Autodesk Fusion 360 part; units mm, degrees
note: some values were not read from the file. Set by a fixed rule: which sketch regions a step uses.
(part 4 of 5)
  line L709 (-95.6805, -65.95) -> (-95.5765, -65.8721)
  line L710 (-95.5765, -65.8721) -> (-95.4672, -65.8024)
  line L711 (-95.4672, -65.8024) -> (-95.3531, -65.7412)
  line L712 (-95.3531, -65.7412) -> (-95.2348, -65.6887)
  line L713 (-95.2348, -65.6887) -> (-95.1128, -65.6452)
  line L714 (-95.1128, -65.6452) -> (-94.9876, -65.6109)
  line L715 (-94.9876, -65.6109) -> (-94.8598, -65.586)
  line L716 (-94.8598, -65.586) -> (-94.7298, -65.5709)
  line L717 (-94.7298, -65.5709) -> (-94.5983, -65.5659)
  line L718 (-94.5983, -65.5659) -> (-94.4542, -65.5719)
  line L719 (-94.4542, -65.5719) -> (-94.3095, -65.5904)
  line L720 (-94.3095, -65.5904) -> (-94.1649, -65.6216)
  line L721 (-94.1649, -65.6216) -> (-94.0212, -65.666)
  line L722 (-94.0212, -65.666) -> (-93.8589, -65.7335)
  line L723 (-93.8589, -65.7335) -> (-93.7072, -65.8154)
  line L724 (-93.7072, -65.8154) -> (-93.5666, -65.9106)
  line L725 (-93.5666, -65.9106) -> (-93.4375, -66.0181)
  line L726 (-93.4375, -66.0181) -> (-93.3205, -66.1366)
  line L727 (-93.3205, -66.1366) -> (-93.2162, -66.2652)
  line L728 (-93.2162, -66.2652) -> (-93.125, -66.4027)
  line L729 (-93.125, -66.4027) -> (-93.0475, -66.548)
  line L730 (-93.0475, -66.548) -> (-92.9842, -66.7)
  line L731 (-92.9842, -66.7) -> (-92.9356, -66.8576)
  line L732 (-92.9356, -66.8576) -> (-92.9022, -67.0198)
  line L733 (-92.9022, -67.0198) -> (-92.8846, -67.1853)
  line L734 (-92.8846, -67.1853) -> (-92.8836, -67.3531)
  line L735 (-92.8836, -67.3531) -> (-92.8991, -67.5221)
  line L736 (-92.8991, -67.5221) -> (-92.9319, -67.6912)
  line L737 (-92.9319, -67.6912) -> (-92.9826, -67.8593)
  line L738 (-92.9826, -67.8593) -> (-95.8873, -75.988)
  line L739 (-95.8873, -75.988) -> (-94.5986, -75.988)
  line L740 (-94.5986, -75.988) -> (-94.479, -75.994)
  line L741 (-94.479, -75.994) -> (-94.3628, -76.0117)
  line L742 (-94.3628, -76.0117) -> (-94.2506, -76.0405)
  line L743 (-94.2506, -76.0405) -> (-94.1431, -76.0799)
  line L744 (-94.1431, -76.0799) -> (-94.0408, -76.1291)
  line L745 (-94.0408, -76.1291) -> (-93.9443, -76.1877)
  line L746 (-93.9443, -76.1877) -> (-93.8542, -76.2551)
  line L747 (-93.8542, -76.2551) -> (-93.7711, -76.3306)
  line L748 (-93.7711, -76.3306) -> (-93.6955, -76.4137)
  line L749 (-93.6955, -76.4137) -> (-93.6281, -76.5038)
  line L750 (-93.6281, -76.5038) -> (-93.5695, -76.6003)
  line L751 (-93.5695, -76.6003) -> (-93.5202, -76.7026)
  line L752 (-93.5202, -76.7026) -> (-93.4808, -76.8102)
  line L753 (-93.4808, -76.8102) -> (-93.4519, -76.9224)
  line L754 (-93.4519, -76.9224) -> (-93.4342, -77.0387)
  line L755 (-93.4342, -77.0387) -> (-93.4282, -77.1585)
  line L756 (-93.4282, -77.1585) -> (-93.4342, -77.2781)
  line L757 (-93.4342, -77.2781) -> (-93.4519, -77.3943)
  line L758 (-93.4519, -77.3943) -> (-93.4808, -77.5065)
  line L759 (-93.4808, -77.5065) -> (-93.5202, -77.614)
  line L760 (-93.5202, -77.614) -> (-93.5695, -77.7163)
  line L761 (-93.5695, -77.7163) -> (-93.6281, -77.8128)
  line L762 (-93.6281, -77.8128) -> (-93.6955, -77.9029)
  line L763 (-93.6955, -77.9029) -> (-93.7711, -77.986)
  line L764 (-93.7711, -77.986) -> (-93.8542, -78.0616)
  line L765 (-93.8542, -78.0616) -> (-93.9443, -78.129)
  line L766 (-93.9443, -78.129) -> (-94.0408, -78.1876)
  line L767 (-94.0408, -78.1876) -> (-94.1431, -78.2369)
  line L768 (-94.1431, -78.2369) -> (-94.2506, -78.2763)
  line L769 (-94.2506, -78.2763) -> (-94.3628, -78.3051)
  line L770 (-94.3628, -78.3051) -> (-94.479, -78.3229)
  line L771 (-94.479, -78.3229) -> (-94.5986, -78.3289)
  line L772 (-94.5986, -78.3289) -> (-98.0467, -78.3289)
  line L773 (-98.0467, -78.3289) -> (-98.1858, -78.3189)
  line L774 (-98.1858, -78.3189) -> (-98.3201, -78.293)
  line L775 (-98.3201, -78.293) -> (-98.4083, -78.3)
  line L776 (-98.4083, -78.3) -> (-98.4224, -78.299)
  line L777 (-98.4224, -78.299) -> (-98.606, -78.291)
  line L778 (-98.606, -78.291) -> (-98.7865, -78.2694)
  line L779 (-98.7865, -78.2694) -> (-98.9634, -78.2348)
  line L780 (-98.9634, -78.2348) -> (-99.1359, -78.1876)
  line L781 (-99.1359, -78.1876) -> (-99.3035, -78.1282)
  line L782 (-99.3035, -78.1282) -> (-99.4654, -78.0571)
  line L783 (-99.4654, -78.0571) -> (-99.6212, -77.9746)
  line L784 (-99.6212, -77.9746) -> (-99.7701, -77.8812)
  line L785 (-99.7701, -77.8812) -> (-99.9116, -77.7774)
  line L786 (-99.9116, -77.7774) -> (-100.045, -77.6636)
  line L787 (-100.045, -77.6636) -> (-100.1696, -77.5402)
  line L788 (-100.1696, -77.5402) -> (-100.285, -77.4076)
  line L789 (-100.285, -77.4076) -> (-100.3903, -77.2662)
  line L790 (-100.3903, -77.2662) -> (-100.4851, -77.1166)
  line L791 (-100.4851, -77.1166) -> (-100.5686, -76.959)
  line L792 (-100.5686, -76.959) -> (-100.6403, -76.7941)
  line L793 (-100.6403, -76.7941) -> (-102.7545, -71.7649)
  line L794 (-102.7545, -71.7649) -> (-104.868, -76.793)
  line L795 (-104.868, -76.793) -> (-104.9397, -76.9586)
  line L796 (-104.9397, -76.9586) -> (-105.0233, -77.1168)
  line L797 (-105.0233, -77.1168) -> (-105.1182, -77.267)
  line L798 (-105.1182, -77.267) -> (-105.2238, -77.4089)
  line L799 (-105.2238, -77.4089) -> (-105.3395, -77.542)
  line L800 (-105.3395, -77.542) -> (-105.4645, -77.6658)
  line L801 (-105.4645, -77.6658) -> (-105.5984, -77.78)
  line L802 (-105.5984, -77.78) -> (-105.7403, -77.8841)
  line L803 (-105.7403, -77.8841) -> (-105.8898, -77.9776)
  line L804 (-105.8898, -77.9776) -> (-106.0461, -78.0602)
  line L805 (-106.0461, -78.0602) -> (-106.2087, -78.1313)
  line L806 (-106.2087, -78.1313) -> (-106.3768, -78.1906)
  line L807 (-106.3768, -78.1906) -> (-106.5499, -78.2376)
  line L808 (-106.5499, -78.2376) -> (-106.7273, -78.2719)
  line L809 (-106.7273, -78.2719) -> (-106.9084, -78.293)
  line L810 (-106.9084, -78.293) -> (-107.0926, -78.3)
  line L811 (-107.0926, -78.3) -> (-107.0996, -78.3008)
  line L812 (-107.0996, -78.3008) -> (-107.288, -78.2938)
  line L813 (-107.288, -78.2938) -> (-107.4733, -78.2722)
  line L814 (-107.4733, -78.2722) -> (-107.6547, -78.2368)
  line L815 (-107.6547, -78.2368) -> (-107.8316, -78.1881)
  line L816 (-107.8316, -78.1881) -> (-108.0032, -78.1266)
  line L817 (-108.0032, -78.1266) -> (-108.169, -78.0527)
  line L818 (-108.169, -78.0527) -> (-108.3282, -77.9669)
  line L819 (-108.3282, -77.9669) -> (-108.4802, -77.8696)
  line L820 (-108.4802, -77.8696) -> (-108.6242, -77.7613)
  line L821 (-108.6242, -77.7613) -> (-108.7595, -77.6426)
  line L822 (-108.7595, -77.6426) -> (-108.8856, -77.5138)
  line L823 (-108.8856, -77.5138) -> (-109.0017, -77.3755)
  line L824 (-109.0017, -77.3755) -> (-109.1071, -77.2281)
  line L825 (-109.1071, -77.2281) -> (-109.2012, -77.0721)
  line L826 (-109.2012, -77.0721) -> (-109.2832, -76.9079)
  line L827 (-109.2832, -76.9079) -> (-109.3525, -76.7362)
  line L828 (-109.3525, -76.7362) -> (-112.5246, -67.8603)
  line L829 (-112.5246, -67.8603) -> (-112.5744, -67.6917)
  line L830 (-112.5744, -67.6917) -> (-112.6072, -67.5226)
  line L831 (-112.6072, -67.5226) -> (-112.6227, -67.3536)
  line L832 (-123.9451, -66.3953) -> (-123.8658, -66.5621)
  line L833 (-123.8658, -66.5621) -> (-123.8011, -66.7379)
  line L834 (-123.8011, -66.7379) -> (-123.7502, -66.9213)
  line L835 (-123.7502, -66.9213) -> (-123.7123, -67.1111)
  line L836 (-123.7123, -67.1111) -> (-123.6866, -67.3062)
  line L837 (-123.6866, -67.3062) -> (-123.6722, -67.5054)
  line L838 (-123.6722, -67.5054) -> (-123.4156, -67.2357)
  line L839 (-123.4156, -67.2357) -> (-123.1539, -66.9883)
  line L840 (-123.1539, -66.9883) -> (-122.887, -66.7624)
  line L841 (-122.887, -66.7624) -> (-122.6149, -66.5573)
  line L842 (-122.6149, -66.5573) -> (-122.3375, -66.3725)
  line L843 (-122.3375, -66.3725) -> (-122.0547, -66.2072)
  line L844 (-122.0547, -66.2072) -> (-121.7664, -66.0609)
  line L845 (-121.7664, -66.0609) -> (-121.4727, -65.9327)
  line L846 (-121.4727, -65.9327) -> (-121.1733, -65.8221)
  line L847 (-121.1733, -65.8221) -> (-120.8684, -65.7284)
  line L848 (-120.8684, -65.7284) -> (-120.5577, -65.6509)
  line L849 (-120.5577, -65.6509) -> (-120.2412, -65.589)
  line L850 (-120.2412, -65.589) -> (-119.9188, -65.542)
  line L851 (-119.9188, -65.542) -> (-119.5906, -65.5093)
  line L852 (-119.5906, -65.5093) -> (-119.2563, -65.4903)
  line L853 (-119.2563, -65.4903) -> (-118.916, -65.4843)
  line L854 (-118.916, -65.4843) -> (-118.7311, -65.4883)
  line L855 (-118.7311, -65.4883) -> (-118.5467, -65.5002)
  line L856 (-118.5467, -65.5002) -> (-118.3631, -65.5198)
  line L857 (-118.3631, -65.5198) -> (-118.1807, -65.547)
  line L858 (-118.1807, -65.547) -> (-117.9999, -65.5818)
  line L859 (-117.9999, -65.5818) -> (-117.8209, -65.624)
  line L860 (-117.8209, -65.624) -> (-117.6443, -65.6736)
  line L861 (-117.6443, -65.6736) -> (-117.4702, -65.7305)
  line L862 (-117.4702, -65.7305) -> (-117.2991, -65.7945)
  line L863 (-117.2991, -65.7945) -> (-117.1313, -65.8656)
  line L864 (-117.1313, -65.8656) -> (-116.9672, -65.9437)
  line L865 (-116.9672, -65.9437) -> (-116.8071, -66.0287)
  line L866 (-116.8071, -66.0287) -> (-116.6513, -66.1205)
  line L867 (-116.6513, -66.1205) -> (-116.5003, -66.219)
  line L868 (-116.5003, -66.219) -> (-116.3544, -66.3241)
  line L869 (-116.3544, -66.3241) -> (-116.2139, -66.4357)
  line L870 (-116.2139, -66.4357) -> (-116.0791, -66.5536)
  line L871 (-116.0791, -66.5536) -> (-115.9505, -66.6779)
  line L872 (-115.9505, -66.6779) -> (-115.8284, -66.8085)
  line L873 (-115.8284, -66.8085) -> (-115.7132, -66.9451)
  line L874 (-115.7132, -66.9451) -> (-115.6051, -67.0878)
  line L875 (-115.6051, -67.0878) -> (-115.5046, -67.2364)
  line L876 (-115.5046, -67.2364) -> (-115.412, -67.3908)
  line L877 (-115.412, -67.3908) -> (-115.3276, -67.551)
  line L878 (-115.3276, -67.551) -> (-115.2518, -67.7168)
  line L879 (-115.2518, -67.7168) -> (-115.185, -67.8882)
  line L880 (-115.185, -67.8882) -> (-115.1275, -68.065)
  line L881 (-115.1275, -68.065) -> (-115.0797, -68.2472)
  line L882 (-115.0797, -68.2472) -> (-115.0419, -68.4346)
  line L883 (-115.0419, -68.4346) -> (-115.0145, -68.6272)
  line L884 (-115.0145, -68.6272) -> (-114.9978, -68.8249)
  line L885 (-114.9978, -68.8249) -> (-114.9918, -69.0276)
  line L886 (-114.9918, -69.0276) -> (-114.9978, -69.2913)
  line L887 (-114.9978, -69.2913) -> (-115.0167, -69.5432)
  line L888 (-115.0167, -69.5432) -> (-115.0478, -69.7836)
  line L889 (-115.0478, -69.7836) -> (-115.0907, -70.0127)
  line L890 (-115.0907, -70.0127) -> (-115.1452, -70.2308)
  line L891 (-115.1452, -70.2308) -> (-115.2109, -70.4382)
  line L892 (-115.2109, -70.4382) -> (-115.2876, -70.6352)
  line L893 (-115.2876, -70.6352) -> (-115.3749, -70.8221)
  line L894 (-115.3749, -70.8221) -> (-115.4725, -70.9992)
  line L895 (-115.4725, -70.9992) -> (-115.5801, -71.1668)
  line L896 (-115.5801, -71.1668) -> (-115.6974, -71.3251)
  line L897 (-115.6974, -71.3251) -> (-115.8241, -71.4744)
  line L898 (-115.8241, -71.4744) -> (-115.9599, -71.6151)
  line L899 (-115.9599, -71.6151) -> (-116.1043, -71.7474)
  line L900 (-116.1043, -71.7474) -> (-116.2573, -71.8716)
  line L901 (-116.2573, -71.8716) -> (-116.4183, -71.9879)
  line L902 (-116.4183, -71.9879) -> (-116.5871, -72.0968)
  line L903 (-116.5871, -72.0968) -> (-116.7634, -72.1984)
  line L904 (-116.7634, -72.1984) -> (-116.9469, -72.2931)
  line L905 (-116.9469, -72.2931) -> (-117.1373, -72.3811)
  line L906 (-117.1373, -72.3811) -> (-117.3342, -72.4627)
  line L907 (-117.3342, -72.4627) -> (-117.5374, -72.5382)
  line L908 (-117.5374, -72.5382) -> (-117.9611, -72.6722)
  line L909 (-117.9611, -72.6722) -> (-118.406, -72.7853)
  line L910 (-118.406, -72.7853) -> (-118.8696, -72.8798)
  line L911 (-118.8696, -72.8798) -> (-119.3494, -72.958)
  line L912 (-119.3494, -72.958) -> (-119.8428, -73.0222)
  line L913 (-119.8428, -73.0222) -> (-119.9037, -73.0252)
  line L914 (-119.9037, -73.0252) -> (-120.0568, -73.0282)
  line L915 (-120.0568, -73.0282) -> (-120.2756, -73.0155)
  line L916 (-120.2756, -73.0155) -> (-120.4012, -72.9983)
  line L917 (-120.4012, -72.9983) -> (-120.5332, -72.9709)
  line L918 (-120.5332, -72.9709) -> (-120.6684, -72.9315)
  line L919 (-120.6684, -72.9315) -> (-120.8032, -72.878)
  line L920 (-120.8032, -72.878) -> (-120.9345, -72.8083)
  line L921 (-120.9345, -72.8083) -> (-121.0588, -72.7204)
  line L922 (-121.0588, -72.7204) -> (-121.1729, -72.6123)
  line L923 (-121.1729, -72.6123) -> (-121.2734, -72.482)
  line L924 (-121.2734, -72.482) -> (-121.357, -72.3274)
  line L925 (-121.357, -72.3274) -> (-121.4203, -72.1465)
  line L926 (-121.4203, -72.1465) -> (-121.4581, -71.9616)
  line L927 (-121.4581, -71.9616) -> (-121.4694, -71.7956)
  line L928 (-121.4694, -71.7956) -> (-121.4576, -71.6475)
  line L929 (-121.4576, -71.6475) -> (-121.4259, -71.5165)
  line L930 (-121.4259, -71.5165) -> (-121.3776, -71.4014)
  line L931 (-121.3776, -71.4014) -> (-121.3161, -71.3013)
  line L932 (-121.3161, -71.3013) -> (-121.2446, -71.2152)
  line L933 (-121.2446, -71.2152) -> (-121.1665, -71.1421)
  line L934 (-121.1665, -71.1421) -> (-121.0851, -71.081)
  line L935 (-121.0851, -71.081) -> (-121.0036, -71.031)
  line L936 (-121.0036, -71.031) -> (-120.8538, -70.9601)
  line L937 (-120.8538, -70.9601) -> (-120.7434, -70.9215)
  line L938 (-120.7434, -70.9215) -> (-120.6989, -70.9072)
  line L939 (-120.6989, -70.9072) -> (-120.4347, -70.8642)
  line L940 (-120.4347, -70.8642) -> (-120.1863, -70.8151)
  line L941 (-120.1863, -70.8151) -> (-119.9539, -70.7594)
  line L942 (-119.9539, -70.7594) -> (-119.7376, -70.6965)
  line L943 (-119.7376, -70.6965) -> (-119.5376, -70.6259)
  line L944 (-119.5376, -70.6259) -> (-119.354, -70.5472)
  line L945 (-119.354, -70.5472) -> (-119.1872, -70.4597)
  line L946 (-119.1872, -70.4597) -> (-119.0371, -70.363)
  line L947 (-119.0371, -70.363) -> (-118.9041, -70.2565)
  line L948 (-118.9041, -70.2565) -> (-118.7882, -70.1398)
  line L949 (-118.7882, -70.1398) -> (-118.6897, -70.0123)
  line L950 (-118.6897, -70.0123) -> (-118.6087, -69.8735)
  line L951 (-118.6087, -69.8735) -> (-118.5454, -69.7228)
  line L952 (-118.5454, -69.7228) -> (-118.5, -69.5598)
  line L953 (-118.5, -69.5598) -> (-118.4726, -69.384)
  line L954 (-118.4726, -69.384) -> (-118.4636, -69.1947)
  line L955 (-118.4636, -69.1947) -> (-118.4726, -69.0494)
  line L956 (-118.4726, -69.0494) -> (-118.4981, -68.9082)
  line L957 (-118.4981, -68.9082) -> (-118.54, -68.7717)
  line L958 (-118.54, -68.7717) -> (-118.5979, -68.6408)
  line L959 (-118.5979, -68.6408) -> (-118.6715, -68.5162)
  line L960 (-118.6715, -68.5162) -> (-118.7602, -68.3986)
  line L961 (-118.7602, -68.3986) -> (-118.8637, -68.2887)
  line L962 (-118.8637, -68.2887) -> (-118.9816, -68.1873)
  line L963 (-118.9816, -68.1873) -> (-119.1134, -68.0951)
  line L964 (-119.1134, -68.0951) -> (-119.2587, -68.0128)
  line L965 (-119.2587, -68.0128) -> (-119.417, -67.9412)
  line L966 (-119.417, -67.9412) -> (-119.5881, -67.881)
  line L967 (-119.5881, -67.881) -> (-119.7714, -67.8329)
  line L968 (-119.7714, -67.8329) -> (-119.9665, -67.7976)
  line L969 (-119.9665, -67.7976) -> (-120.173, -67.7759)
  line L970 (-120.173, -67.7759) -> (-120.3905, -67.7689)
  line L971 (-120.3905, -67.7689) -> (-120.7384, -67.7832)
  line L972 (-120.7384, -67.7832) -> (-121.0683, -67.8246)
  line L973 (-121.0683, -67.8246) -> (-121.3798, -67.8915)
  line L974 (-121.3798, -67.8915) -> (-121.6721, -67.9822)
  line L975 (-121.6721, -67.9822) -> (-121.9446, -68.0949)
  line L976 (-121.9446, -68.0949) -> (-122.1967, -68.2279)
  line L977 (-122.1967, -68.2279) -> (-122.4278, -68.3793)
  line L978 (-122.4278, -68.3793) -> (-122.6372, -68.5476)
  line L979 (-122.6372, -68.5476) -> (-122.8244, -68.7308)
  line L980 (-122.8244, -68.7308) -> (-122.9886, -68.9274)
  line L981 (-122.9886, -68.9274) -> (-123.1293, -69.1355)
  line L982 (-123.1293, -69.1355) -> (-123.2458, -69.3535)
  line L983 (-123.2458, -69.3535) -> (-123.3375, -69.5795)
  line L984 (-123.3375, -69.5795) -> (-123.4038, -69.8118)
  line L985 (-123.4038, -69.8118) -> (-123.444, -70.0488)
  line L986 (-123.444, -70.0488) -> (-123.4576, -70.2886)
  line L987 (-123.4576, -70.2886) -> (-123.4576, -74.5459)
  line L988 (-123.4576, -74.5459) -> (-123.4458, -74.7233)
  line L989 (-123.4458, -74.7233) -> (-123.4114, -74.8818)
  line L990 (-123.4114, -74.8818) -> (-123.3556, -75.0225)
  line L991 (-123.3556, -75.0225) -> (-123.2797, -75.1463)
  line L992 (-123.2797, -75.1463) -> (-123.185, -75.2544)
  line L993 (-123.185, -75.2544) -> (-123.0728, -75.3477)
  line L994 (-123.0728, -75.3477) -> (-122.9443, -75.4272)
  line L995 (-122.9443, -75.4272) -> (-122.801, -75.494)
  line L996 (-122.801, -75.494) -> (-122.6439, -75.5491)
  line L997 (-122.6439, -75.5491) -> (-122.4745, -75.5935)
  line L998 (-122.4745, -75.5935) -> (-122.294, -75.6283)
  line L999 (-122.294, -75.6283) -> (-122.1036, -75.6545)
  line L1000 (-122.1036, -75.6545) -> (-121.6987, -75.685)
  line L1001 (-121.6987, -75.685) -> (-121.2699, -75.693)
  line L1002 (-121.2699, -75.693) -> (-120.0878, -75.693)
  line L1003 (-120.0878, -75.693) -> (-116.8006, -75.1659)
  line L1004 (-116.8006, -75.1659) -> (-116.6326, -75.1503)
  line L1005 (-116.6326, -75.1503) -> (-116.4755, -75.1533)
  line L1006 (-116.4755, -75.1533) -> (-116.3294, -75.1745)
  line L1007 (-116.3294, -75.1745) -> (-116.1941, -75.2121)
  line L1008 (-116.1941, -75.2121) -> (-116.0697, -75.2646)
  line L1009 (-116.0697, -75.2646) -> (-115.9561, -75.3306)
  line L1010 (-115.9561, -75.3306) -> (-115.8534, -75.4086)
  line L1011 (-115.8534, -75.4086) -> (-115.7616, -75.4972)
  line L1012 (-115.7616, -75.4972) -> (-115.6806, -75.595)
  line L1013 (-115.6806, -75.595) -> (-115.6104, -75.7006)
  line L1014 (-115.6104, -75.7006) -> (-115.551, -75.8125)
  line L1015 (-115.551, -75.8125) -> (-115.5025, -75.9293)
  line L1016 (-115.5025, -75.9293) -> (-115.4648, -76.0496)
  line L1017 (-115.4648, -76.0496) -> (-115.4379, -76.172)
  line L1018 (-115.4379, -76.172) -> (-115.4217, -76.295)
  line L1019 (-115.4217, -76.295) -> (-115.4167, -76.4171)
  line L1020 (-115.4167, -76.4171) -> (-115.4247, -76.5699)
  line L1021 (-115.4247, -76.5699) -> (-115.447, -76.7125)
  line L1022 (-115.447, -76.7125) -> (-115.483, -76.8451)
  line L1023 (-115.483, -76.8451) -> (-115.5319, -76.9681)
  line L1024 (-115.5319, -76.9681) -> (-115.5928, -77.0817)
  line L1025 (-115.5928, -77.0817) -> (-115.6648, -77.1863)
  line L1026 (-115.6648, -77.1863) -> (-115.747, -77.2821)
  line L1027 (-115.747, -77.2821) -> (-115.8386, -77.3695)
  line L1028 (-115.8386, -77.3695) -> (-115.9387, -77.4488)
  line L1029 (-115.9387, -77.4488) -> (-116.0463, -77.5203)
  line L1030 (-116.0463, -77.5203) -> (-116.1605, -77.5843)
  line L1031 (-116.1605, -77.5843) -> (-116.2806, -77.641)
  line L1032 (-116.2806, -77.641) -> (-116.4057, -77.6908)
  line L1033 (-116.4057, -77.6908) -> (-116.5347, -77.734)
  line L1034 (-116.5347, -77.734) -> (-116.8014, -77.8018)
  line L1035 (-116.8014, -77.8018) -> (-119.8307, -78.2988)
  line L1036 (-119.8307, -78.2988) -> (-120.6654, -78.2888)
  line L1037 (-120.6654, -78.2888) -> (-121.4511, -78.2582)
  line L1038 (-121.4511, -78.2582) -> (-122.1871, -78.2057)
  line L1039 (-122.1871, -78.2057) -> (-122.8727, -78.1301)
  line L1040 (-122.8727, -78.1301) -> (-123.1964, -78.0833)
  line L1041 (-123.1964, -78.0833) -> (-123.5073, -78.0302)
  line L1042 (-123.5073, -78.0302) -> (-123.8053, -77.9707)
  line L1043 (-123.8053, -77.9707) -> (-124.0902, -77.9047)
  line L1044 (-124.0902, -77.9047) -> (-124.3621, -77.832)
  line L1045 (-124.3621, -77.832) -> (-124.6208, -77.7524)
  line L1046 (-124.6208, -77.7524) -> (-124.8662, -77.6658)
  line L1047 (-124.8662, -77.6658) -> (-125.0983, -77.5721)
  line L1048 (-125.0983, -77.5721) -> (-125.317, -77.4711)
  line L1049 (-125.317, -77.4711) -> (-125.5222, -77.3626)
  line L1050 (-125.5222, -77.3626) -> (-125.7138, -77.2464)
  line L1051 (-125.7138, -77.2464) -> (-125.8917, -77.1225)
  line L1052 (-125.8917, -77.1225) -> (-126.0559, -76.9907)
  line L1053 (-126.0559, -76.9907) -> (-126.2062, -76.8507)
  line L1054 (-126.2062, -76.8507) -> (-126.3426, -76.7026)
  line L1055 (-126.3426, -76.7026) -> (-126.465, -76.546)
  line L1056 (-126.465, -76.546) -> (-126.5733, -76.3809)
  line L1057 (-126.5733, -76.3809) -> (-126.6674, -76.2071)
  line L1058 (-126.6674, -76.2071) -> (-126.7473, -76.0244)
  line L1059 (-126.7473, -76.0244) -> (-126.8129, -75.8328)
  line L1060 (-126.8129, -75.8328) -> (-126.864, -75.6319)
  line L1061 (-126.864, -75.6319) -> (-126.9006, -75.4218)
  line L1062 (-126.9006, -75.4218) -> (-126.9226, -75.2022)
  line L1063 (-126.9226, -75.2022) -> (-126.9296, -74.973)
  line L1064 (-126.9296, -74.973) -> (-126.9296, -69.1468)
  line L1065 (-126.9296, -69.1468) -> (-126.9332, -68.8866)
  line L1066 (-126.9332, -68.8866) -> (-126.9445, -68.6517)
  line L1067 (-126.9445, -68.6517) -> (-126.9621, -68.439)
  line L1068 (-126.9621, -68.439) -> (-126.9849, -68.2467)
  line L1069 (-126.9849, -68.2467) -> (-127.0421, -67.9152)
  line L1070 (-127.0421, -67.9152) -> (-127.1076, -67.6416)
  line L1071 (-127.1076, -67.6416) -> (-127.1731, -67.4104)
  line L1072 (-127.1731, -67.4104) -> (-127.2303, -67.206)
  line L1073 (-127.2303, -67.206) -> (-127.2707, -67.0128)
  line L1074 (-127.2707, -67.0128) -> (-127.286, -66.8152)
  line L1075 (-127.286, -66.8152) -> (-127.278, -66.671)
  line L1076 (-127.278, -66.671) -> (-127.2532, -66.5328)
  line L1077 (-127.2532, -66.5328) -> (-127.213, -66.401)
  line L1078 (-127.213, -66.401) -> (-127.1583, -66.2762)
  line L1079 (-127.1583, -66.2762) -> (-127.0901, -66.1588)
  line L1080 (-127.0901, -66.1588) -> (-127.0093, -66.0492)
  line L1081 (-127.0093, -66.0492) -> (-126.9169, -65.9479)
  line L1082 (-126.9169, -65.9479) -> (-126.8138, -65.8554)
  line L1083 (-126.8138, -65.8554) -> (-126.7009, -65.772)
  line L1084 (-126.7009, -65.772) -> (-126.5793, -65.6983)
  line L1085 (-126.5793, -65.6983) -> (-126.4497, -65.6347)
  line L1086 (-126.4497, -65.6347) -> (-126.3132, -65.5816)
  line L1087 (-126.3132, -65.5816) -> (-126.1707, -65.5395)
  line L1088 (-126.1707, -65.5395) -> (-126.0231, -65.5089)
  line L1089 (-126.0231, -65.5089) -> (-125.8714, -65.4901)
  line L1090 (-125.8714, -65.4901) -> (-125.7165, -65.4841)
  line L1091 (-125.7165, -65.4841) -> (-125.4473, -65.4949)
  line L1092 (-125.4473, -65.4949) -> (-125.2007, -65.5269)
  line L1093 (-125.2007, -65.5269) -> (-124.9758, -65.5788)
  line L1094 (-124.9758, -65.5788) -> (-124.772, -65.6493)
  line L1095 (-124.772, -65.6493) -> (-124.5884, -65.7372)
  line L1096 (-124.5884, -65.7372) -> (-124.4241, -65.8412)
  line L1097 (-124.4241, -65.8412) -> (-124.2785, -65.9603)
  line L1098 (-124.2785, -65.9603) -> (-124.1506, -66.0932)
  line L1099 (-124.1506, -66.0932) -> (-124.0398, -66.2386)
  line L1100 (-124.0398, -66.2386) -> (-123.9451, -66.3953)
  line L1101 (-68.7045, -83.0443) -> (-68.801, -83.1029)
  line L1102 (-68.801, -83.1029) -> (-68.9034, -83.1522)
  line L1103 (-68.9034, -83.1522) -> (-69.0109, -83.1916)
  line L1104 (-69.0109, -83.1916) -> (-69.1231, -83.2204)
  line L1105 (-69.1231, -83.2204) -> (-69.2394, -83.2381)
  line L1106 (-69.2394, -83.2381) -> (-69.3591, -83.2441)
  line L1107 (-69.3591, -83.2441) -> (-71.2172, -83.2441)
  line L1108 (-71.2172, -83.2441) -> (-71.343, -83.2371)
  line L1109 (-71.343, -83.2371) -> (-71.4648, -83.217)
  line L1110 (-71.4648, -83.217) -> (-71.6462, -83.2032)
  line L1111 (-71.6462, -83.2032) -> (-71.8185, -83.1765)
  line L1112 (-71.8185, -83.1765) -> (-71.9818, -83.1371)
  line L1113 (-71.9818, -83.1371) -> (-72.1359, -83.085)
  line L1114 (-72.1359, -83.085) -> (-72.2803, -83.0202)
  line L1115 (-72.2803, -83.0202) -> (-72.4145, -82.9429)
  line L1116 (-72.4145, -82.9429) -> (-72.538, -82.853)
  line L1117 (-72.538, -82.853) -> (-72.6504, -82.7506)
  line L1118 (-72.6504, -82.7506) -> (-72.7513, -82.6359)
  line L1119 (-72.7513, -82.6359) -> (-72.8402, -82.5087)
  line L1120 (-72.8402, -82.5087) -> (-72.9166, -82.3692)
  line L1121 (-72.9166, -82.3692) -> (-72.9802, -82.2175)
  line L1122 (-72.9802, -82.2175) -> (-73.0304, -82.0535)
  line L1123 (-73.0304, -82.0535) -> (-73.0668, -81.8773)
  line L1124 (-73.0668, -81.8773) -> (-73.089, -81.689)
  line L1125 (-73.089, -81.689) -> (-73.096, -81.4885)
  line L1126 (-73.096, -81.4885) -> (-73.096, -67.2204)
  line L1127 (-73.096, -67.2204) -> (-73.088, -67.0129)
  line L1128 (-73.088, -67.0129) -> (-73.0643, -66.8183)
  line L1129 (-73.0643, -66.8183) -> (-73.0254, -66.6366)
  line L1130 (-73.0254, -66.6366) -> (-72.9718, -66.468)
  line L1131 (-72.9718, -66.468) -> (-72.904, -66.3124)
  line L1132 (-72.904, -66.3124) -> (-72.8225, -66.17)
  line L1133 (-72.8225, -66.17) -> (-72.7278, -66.0408)
  line L1134 (-72.7278, -66.0408) -> (-72.6203, -65.9249)
  line L1135 (-72.6203, -65.9249) -> (-72.5006, -65.8224)
  line L1136 (-72.5006, -65.8224) -> (-72.3691, -65.7333)
  line L1137 (-72.3691, -65.7333) -> (-72.2263, -65.6578)
  line L1138 (-72.2263, -65.6578) -> (-72.0727, -65.5958)
  line L1139 (-72.0727, -65.5958) -> (-71.9088, -65.5475)
  line L1140 (-71.9088, -65.5475) -> (-71.7351, -65.5129)
  line L1141 (-71.7351, -65.5129) -> (-71.5521, -65.492)
  line L1142 (-71.5521, -65.492) -> (-71.3602, -65.485)
  line L1143 (-71.3602, -65.485) -> (-71.1683, -65.492)
  line L1144 (-71.1683, -65.492) -> (-70.9852, -65.5129)
  line L1145 (-70.9852, -65.5129) -> (-70.8115, -65.5475)
  line L1146 (-70.8115, -65.5475) -> (-70.6475, -65.5958)
  line L1147 (-70.6475, -65.5958) -> (-70.4939, -65.6578)
  line L1148 (-70.4939, -65.6578) -> (-70.3511, -65.7333)
  line L1149 (-70.3511, -65.7333) -> (-70.2196, -65.8224)
  line L1150 (-70.2196, -65.8224) -> (-70.0998, -65.9249)
  line L1151 (-70.0998, -65.9249) -> (-69.9923, -66.0408)
  line L1152 (-69.9923, -66.0408) -> (-69.8975, -66.17)
  line L1153 (-69.8975, -66.17) -> (-69.816, -66.3124)
  line L1154 (-69.816, -66.3124) -> (-69.7482, -66.468)
  line L1155 (-69.7482, -66.468) -> (-69.6946, -66.6366)
  line L1156 (-69.6946, -66.6366) -> (-69.6557, -66.8183)
  line L1157 (-69.6557, -66.8183) -> (-69.632, -67.0129)
  line L1158 (-69.632, -67.0129) -> (-69.624, -67.2204)
  line L1159 (-69.624, -67.2204) -> (-69.624, -80.9033)
  line L1160 (-69.624, -80.9033) -> (-69.3591, -80.9033)
  line L1161 (-69.3591, -80.9033) -> (-69.2394, -80.9093)
  line L1162 (-69.2394, -80.9093) -> (-69.1231, -80.927)
  line L1163 (-69.1231, -80.927) -> (-69.0109, -80.9558)
  line L1164 (-69.0109, -80.9558) -> (-68.9034, -80.9952)
  line L1165 (-68.9034, -80.9952) -> (-68.801, -81.0445)
  line L1166 (-68.801, -81.0445) -> (-68.7045, -81.1031)
  line L1167 (-68.7045, -81.1031) -> (-68.6144, -81.1705)
  line L1168 (-68.6144, -81.1705) -> (-68.5313, -81.246)
  line L1169 (-68.5313, -81.246) -> (-68.4557, -81.3291)
  line L1170 (-68.4557, -81.3291) -> (-68.3883, -81.4192)
  line L1171 (-68.3883, -81.4192) -> (-68.3296, -81.5157)
  line L1172 (-68.3296, -81.5157) -> (-68.2803, -81.618)
  line L1173 (-68.2803, -81.618) -> (-68.2409, -81.7256)
  line L1174 (-68.2409, -81.7256) -> (-68.2121, -81.8379)
  line L1175 (-68.2121, -81.8379) -> (-68.1943, -81.9542)
  line L1176 (-68.1943, -81.9542) -> (-68.1883, -82.0739)
  line L1177 (-68.1883, -82.0739) -> (-68.1943, -82.1936)
  line L1178 (-68.1943, -82.1936) -> (-68.2121, -82.3098)
  line L1179 (-68.2121, -82.3098) -> (-68.2409, -82.4219)
  line L1180 (-68.2409, -82.4219) -> (-68.2803, -82.5294)
  line L1181 (-68.2803, -82.5294) -> (-68.3296, -82.6317)
  line L1182 (-68.3296, -82.6317) -> (-68.3883, -82.7282)
  line L1183 (-68.3883, -82.7282) -> (-68.4557, -82.8183)
  line L1184 (-68.4557, -82.8183) -> (-68.5313, -82.9014)
  line L1185 (-68.5313, -82.9014) -> (-68.6144, -82.9769)
  line L1186 (-68.6144, -82.9769) -> (-68.7045, -83.0443)
  line L1187 (-87.842, -78.5031) -> (-88.063, -78.5303)
  line L1188 (-88.063, -78.5303) -> (-88.3059, -78.5393)
  line L1189 (-88.3059, -78.5393) -> (-88.5487, -78.5303)
  line L1190 (-88.5487, -78.5303) -> (-88.7696, -78.5031)
  line L1191 (-88.7696, -78.5031) -> (-88.9694, -78.4589)
  line L1192 (-88.9694, -78.4589) -> (-89.1489, -78.3988)
  line L1193 (-89.1489, -78.3988) -> (-89.309, -78.3238)
  line L1194 (-89.309, -78.3238) -> (-89.4507, -78.2349)
  line L1195 (-89.4507, -78.2349) -> (-89.5747, -78.1332)
  line L1196 (-89.5747, -78.1332) -> (-89.682, -78.0196)
  line L1197 (-89.682, -78.0196) -> (-89.7734, -77.8951)
  line L1198 (-89.7734, -77.8951) -> (-89.8498, -77.7607)
  line L1199 (-89.8498, -77.7607) -> (-89.912, -77.6175)
  line L1200 (-89.912, -77.6175) -> (-89.961, -77.4665)
  line L1201 (-89.961, -77.4665) -> (-89.9976, -77.3087)
  line L1202 (-89.9976, -77.3087) -> (-90.0226, -77.145)
  line L1203 (-90.0226, -77.145) -> (-90.037, -76.9765)
  line L1204 (-90.037, -76.9765) -> (-90.042, -76.8042)
  line L1205 (-90.042, -76.8042) -> (-90.042, -67.2203)
  line L1206 (-90.042, -67.2203) -> (-90.037, -67.0481)
  line L1207 (-90.037, -67.0481) -> (-90.0226, -66.8796)
  line L1208 (-90.0226, -66.8796) -> (-89.9976, -66.7159)
  line L1209 (-89.9976, -66.7159) -> (-89.961, -66.5581)
  line L1210 (-89.961, -66.5581) -> (-89.912, -66.407)
  line L1211 (-89.912, -66.407) -> (-89.8498, -66.2638)
  line L1212 (-89.8498, -66.2638) -> (-89.7734, -66.1295)
  line L1213 (-89.7734, -66.1295) -> (-89.682, -66.005)
  line L1214 (-89.682, -66.005) -> (-89.5747, -65.8914)
  line L1215 (-89.5747, -65.8914) -> (-89.4507, -65.7896)
  line L1216 (-89.4507, -65.7896) -> (-89.309, -65.7007)
  line L1217 (-89.309, -65.7007) -> (-89.1489, -65.6257)
  line L1218 (-89.1489, -65.6257) -> (-88.9694, -65.5656)
  line L1219 (-88.9694, -65.5656) -> (-88.7696, -65.5214)
  line L1220 (-88.7696, -65.5214) -> (-88.5487, -65.4942)
  line L1221 (-88.5487, -65.4942) -> (-88.3059, -65.4852)
  line L1222 (-88.3059, -65.4852) -> (-88.063, -65.4942)
  line L1223 (-88.063, -65.4942) -> (-87.842, -65.5214)
  line L1224 (-87.842, -65.5214) -> (-87.6422, -65.5656)
  line L1225 (-87.6422, -65.5656) -> (-87.4627, -65.6257)
  line L1226 (-87.4627, -65.6257) -> (-87.3025, -65.7007)
  line L1227 (-87.3025, -65.7007) -> (-87.1608, -65.7896)
  line L1228 (-87.1608, -65.7896) -> (-87.0368, -65.8914)
  line L1229 (-87.0368, -65.8914) -> (-86.9295, -66.005)
  line L1230 (-86.9295, -66.005) -> (-86.8381, -66.1295)
  line L1231 (-86.8381, -66.1295) -> (-86.7617, -66.2638)
  line L1232 (-86.7617, -66.2638) -> (-86.6995, -66.407)
  line L1233 (-86.6995, -66.407) -> (-86.6505, -66.5581)
  line L1234 (-86.6505, -66.5581) -> (-86.6139, -66.7159)
  line L1235 (-86.6139, -66.7159) -> (-86.5888, -66.8796)
  line L1236 (-86.5888, -66.8796) -> (-86.5744, -67.0481)
  line L1237 (-86.5744, -67.0481) -> (-86.5694, -67.2203)
  line L1238 (-86.5694, -67.2203) -> (-86.5694, -76.8042)
  line L1239 (-86.5694, -76.8042) -> (-86.5744, -76.9765)
  line L1240 (-86.5744, -76.9765) -> (-86.5888, -77.145)
  line L1241 (-86.5888, -77.145) -> (-86.6139, -77.3087)
  line L1242 (-86.6139, -77.3087) -> (-86.6505, -77.4665)
  line L1243 (-86.6505, -77.4665) -> (-86.6995, -77.6175)
  line L1244 (-86.6995, -77.6175) -> (-86.7617, -77.7607)
  line L1245 (-86.7617, -77.7607) -> (-86.8381, -77.8951)
  line L1246 (-86.8381, -77.8951) -> (-86.9295, -78.0196)
  line L1247 (-86.9295, -78.0196) -> (-87.0368, -78.1332)
  line L1248 (-87.0368, -78.1332) -> (-87.1608, -78.2349)
  line L1249 (-87.1608, -78.2349) -> (-87.3025, -78.3238)
  line L1250 (-87.3025, -78.3238) -> (-87.4627, -78.3988)
  line L1251 (-87.4627, -78.3988) -> (-87.6422, -78.4589)
  line L1252 (-87.6422, -78.4589) -> (-87.842, -78.5031)
  line L1253 (-82.3396, -78.2162) -> (-82.5031, -78.1971)
  line L1254 (-82.5031, -78.1971) -> (-82.6551, -78.1698)
  line L1255 (-82.6551, -78.1698) -> (-82.7955, -78.134)
  line L1256 (-82.7955, -78.134) -> (-82.9243, -78.0894)
  line L1257 (-82.9243, -78.0894) -> (-83.0413, -78.0357)
  line L1258 (-83.0413, -78.0357) -> (-83.1465, -77.9726)
  line L1259 (-83.1465, -77.9726) -> (-83.2396, -77.8997)
  line L1260 (-83.2396, -77.8997) -> (-83.3207, -77.8168)
  line L1261 (-83.3207, -77.8168) -> (-83.3896, -77.7235)
  line L1262 (-83.3896, -77.7235) -> (-83.4462, -77.6194)
  line L1263 (-83.4462, -77.6194) -> (-83.4904, -77.5044)
  line L1264 (-83.4904, -77.5044) -> (-83.5221, -77.3781)
  line L1265 (-83.5221, -77.3781) -> (-83.5412, -77.2401)
  line L1266 (-83.5412, -77.2401) -> (-83.5472, -77.0903)
  line L1267 (-83.5472, -77.0903) -> (-83.5412, -76.9402)
  line L1268 (-83.5412, -76.9402) -> (-83.5221, -76.8021)
  line L1269 (-83.5221, -76.8021) -> (-83.4904, -76.6757)
  line L1270 (-83.4904, -76.6757) -> (-83.4462, -76.5605)
  line L1271 (-83.4462, -76.5605) -> (-83.3896, -76.4563)
  line L1272 (-83.3896, -76.4563) -> (-83.3207, -76.3628)
  line L1273 (-83.3207, -76.3628) -> (-83.2396, -76.2797)
  line L1274 (-83.2396, -76.2797) -> (-83.1465, -76.2067)
  line L1275 (-83.1465, -76.2067) -> (-83.0413, -76.1434)
  line L1276 (-83.0413, -76.1434) -> (-82.9243, -76.0896)
  line L1277 (-82.9243, -76.0896) -> (-82.7955, -76.0449)
  line L1278 (-82.7955, -76.0449) -> (-82.6551, -76.009)
  line L1279 (-82.6551, -76.009) -> (-82.5031, -75.9816)
  line L1280 (-82.5031, -75.9816) -> (-82.3396, -75.9626)
  line L1281 (-82.3396, -75.9626) -> (-82.1648, -75.9512)
  line L1282 (-82.1648, -75.9512) -> (-81.9787, -75.9472)
  line L1283 (-81.9787, -75.9472) -> (-80.9323, -75.9472)
  line L1284 (-80.9323, -75.9472) -> (-80.9323, -67.1493)
  line L1285 (-80.9323, -67.1493) -> (-80.9243, -66.9418)
  line L1286 (-80.9243, -66.9418) -> (-80.9006, -66.7472)
  line L1287 (-80.9006, -66.7472) -> (-80.8617, -66.5655)
  line L1288 (-80.8617, -66.5655) -> (-80.8081, -66.3968)
  line L1289 (-80.8081, -66.3968) -> (-80.7403, -66.2413)
  line L1290 (-80.7403, -66.2413) -> (-80.6588, -66.0989)
  line L1291 (-80.6588, -66.0989) -> (-80.564, -65.9697)
  line L1292 (-80.564, -65.9697) -> (-80.4565, -65.8538)
  line L1293 (-80.4565, -65.8538) -> (-80.3368, -65.7513)
  line L1294 (-80.3368, -65.7513) -> (-80.2052, -65.6622)
  line L1295 (-80.2052, -65.6622) -> (-80.0624, -65.5866)
  line L1296 (-80.0624, -65.5866) -> (-79.9088, -65.5246)
  line L1297 (-79.9088, -65.5246) -> (-79.7449, -65.4763)
  line L1298 (-79.7449, -65.4763) -> (-79.5712, -65.4417)
  line L1299 (-79.5712, -65.4417) -> (-79.3881, -65.4208)
  line L1300 (-79.3881, -65.4208) -> (-79.1963, -65.4138)
  line L1301 (-79.1963, -65.4138) -> (-79.0043, -65.4208)
  line L1302 (-79.0043, -65.4208) -> (-78.8213, -65.4417)
  line L1303 (-78.8213, -65.4417) -> (-78.6475, -65.4763)
  line L1304 (-78.6475, -65.4763) -> (-78.4836, -65.5246)
  line L1305 (-78.4836, -65.5246) -> (-78.33, -65.5866)
  line L1306 (-78.33, -65.5866) -> (-78.1872, -65.6622)
  line L1307 (-78.1872, -65.6622) -> (-78.0556, -65.7513)
  line L1308 (-78.0556, -65.7513) -> (-77.9359, -65.8538)
  line L1309 (-77.9359, -65.8538) -> (-77.8284, -65.9697)
  line L1310 (-77.8284, -65.9697) -> (-77.7337, -66.0989)
  line L1311 (-77.7337, -66.0989) -> (-77.6522, -66.2413)
  line L1312 (-77.6522, -66.2413) -> (-77.5844, -66.3968)
  line L1313 (-77.5844, -66.3968) -> (-77.5308, -66.5655)
  line L1314 (-77.5308, -66.5655) -> (-77.4919, -66.7472)
  line L1315 (-77.4919, -66.7472) -> (-77.4682, -66.9418)
  line L1316 (-77.4682, -66.9418) -> (-77.4602, -67.1493)
  line L1317 (-77.4602, -67.1493) -> (-77.4602, -75.8859)
  line L1318 (-77.4602, -75.8859) -> (-77.4016, -75.8859)
  line L1319 (-77.4016, -75.8859) -> (-77.2819, -75.8919)
  line L1320 (-77.2819, -75.8919) -> (-77.1657, -75.9096)
  line L1321 (-77.1657, -75.9096) -> (-77.0536, -75.9384)
  line L1322 (-77.0536, -75.9384) -> (-76.9461, -75.9778)
  line L1323 (-76.9461, -75.9778) -> (-76.8438, -76.0271)
  line L1324 (-76.8438, -76.0271) -> (-76.7473, -76.0857)
  line L1325 (-76.7473, -76.0857) -> (-76.6572, -76.1531)
  line L1326 (-76.6572, -76.1531) -> (-76.5741, -76.2287)
  line L1327 (-76.5741, -76.2287) -> (-76.4986, -76.3118)
  line L1328 (-76.4986, -76.3118) -> (-76.4312, -76.4019)
  line L1329 (-76.4312, -76.4019) -> (-76.3726, -76.4984)
  line L1330 (-76.3726, -76.4984) -> (-76.3233, -76.6007)
  line L1331 (-76.3233, -76.6007) -> (-76.2839, -76.7083)
  line L1332 (-76.2839, -76.7083) -> (-76.2551, -76.8206)
  line L1333 (-76.2551, -76.8206) -> (-76.2374, -76.9369)
  line L1334 (-76.2374, -76.9369) -> (-76.2314, -77.0566)
  line L1335 (-76.2314, -77.0566) -> (-76.2374, -77.1762)
  line L1336 (-76.2374, -77.1762) -> (-76.2551, -77.2923)
  line L1337 (-76.2551, -77.2923) -> (-76.2839, -77.4043)
  line L1338 (-76.2839, -77.4043) -> (-76.3233, -77.5118)
  line L1339 (-76.3233, -77.5118) -> (-76.3726, -77.614)
  line L1340 (-76.3726, -77.614) -> (-76.4312, -77.7105)
  line L1341 (-76.4312, -77.7105) -> (-76.4986, -77.8006)
  line L1342 (-76.4986, -77.8006) -> (-76.5741, -77.8837)
  line L1343 (-76.5741, -77.8837) -> (-76.6572, -77.9592)
  line L1344 (-76.6572, -77.9592) -> (-76.7473, -78.0266)
  line L1345 (-76.7473, -78.0266) -> (-76.8438, -78.0852)
  line L1346 (-76.8438, -78.0852) -> (-76.9461, -78.1345)
  line L1347 (-76.9461, -78.1345) -> (-77.0536, -78.1739)
  line L1348 (-77.0536, -78.1739) -> (-77.1657, -78.2028)
  line L1349 (-77.1657, -78.2028) -> (-77.2819, -78.2205)
  line L1350 (-77.2819, -78.2205) -> (-77.4016, -78.2265)
  line L1351 (-77.4016, -78.2265) -> (-77.4602, -78.2265)
  line L1352 (-77.4602, -78.2265) -> (-77.4602, -80.3472)
  line L1353 (-77.4602, -80.3472) -> (-77.4682, -80.5547)
  line L1354 (-77.4682, -80.5547) -> (-77.4919, -80.7493)
  line L1355 (-77.4919, -80.7493) -> (-77.5308, -80.931)
  line L1356 (-77.5308, -80.931) -> (-77.5844, -81.0996)
  line L1357 (-77.5844, -81.0996) -> (-77.6522, -81.2552)
  line L1358 (-77.6522, -81.2552) -> (-77.7337, -81.3976)
  line L1359 (-77.7337, -81.3976) -> (-77.8285, -81.5268)
  line L1360 (-77.8285, -81.5268) -> (-77.936, -81.6427)
  line L1361 (-77.936, -81.6427) -> (-78.0558, -81.7452)
  line L1362 (-78.0558, -81.7452) -> (-78.1873, -81.8343)
  line L1363 (-78.1873, -81.8343) -> (-78.3302, -81.9099)
  line L1364 (-78.3302, -81.9099) -> (-78.4838, -81.9719)
  line L1365 (-78.4838, -81.9719) -> (-78.6478, -82.0202)
  line L1366 (-78.6478, -82.0202) -> (-78.8216, -82.0548)
  line L1367 (-78.8216, -82.0548) -> (-79.0047, -82.0756)
  line L1368 (-79.0047, -82.0756) -> (-79.1967, -82.0826)
  line L1369 (-79.1967, -82.0826) -> (-79.3885, -82.0756)
  line L1370 (-79.3885, -82.0756) -> (-79.5715, -82.0548)
  line L1371 (-79.5715, -82.0548) -> (-79.7451, -82.0202)
  line L1372 (-79.7451, -82.0202) -> (-79.909, -81.9719)
  line L1373 (-79.909, -81.9719) -> (-80.0626, -81.9099)
  line L1374 (-80.0626, -81.9099) -> (-80.2054, -81.8343)
  line L1375 (-80.2054, -81.8343) -> (-80.3369, -81.7452)
  line L1376 (-80.3369, -81.7452) -> (-80.4566, -81.6427)
  line L1377 (-80.4566, -81.6427) -> (-80.5641, -81.5268)
  line L1378 (-80.5641, -81.5268) -> (-80.6588, -81.3976)
  line L1379 (-80.6588, -81.3976) -> (-80.7403, -81.2552)
  line L1380 (-80.7403, -81.2552) -> (-80.8081, -81.0996)
  line L1381 (-80.8081, -81.0996) -> (-80.8617, -80.931)
  line L1382 (-80.8617, -80.931) -> (-80.9006, -80.7493)
  line L1383 (-80.9006, -80.7493) -> (-80.9243, -80.5547)
  line L1384 (-80.9243, -80.5547) -> (-80.9323, -80.3472)
  line L1385 (-80.9323, -80.3472) -> (-80.9323, -78.2305)
  line L1386 (-80.9323, -78.2305) -> (-81.9787, -78.2305)
  line L1387 (-81.9787, -78.2305) -> (-82.1648, -78.2274)
  line L1388 (-82.1648, -78.2274) -> (-82.3396, -78.2162)
  line L1389 (-150.6265, -71.419) -> (-150.4755, -71.5011)
  line L1390 (-150.4755, -71.5011) -> (-150.3406, -71.6057)
  line L1391 (-150.3406, -71.6057) -> (-150.2244, -71.7303)
  line L1392 (-150.2244, -71.7303) -> (-150.1296, -71.8724)
  line L1393 (-150.1296, -71.8724) -> (-150.0587, -72.0296)
  line L1394 (-150.0587, -72.0296) -> (-150.0142, -72.1994)
  line L1395 (-150.0142, -72.1994) -> (-150.0027, -72.2883)
  line L1396 (-150.0027, -72.2883) -> (-149.9987, -72.3794)
  line L1397 (-149.9987, -72.3794) -> (-150.0037, -72.487)
  line L1398 (-150.0037, -72.487) -> (-150.0197, -72.5915)
  line L1399 (-150.0197, -72.5915) -> (-150.0457, -72.6924)
  line L1400 (-150.0457, -72.6924) -> (-150.0811, -72.7892)
  line L1401 (-150.0811, -72.7892) -> (-150.1255, -72.8813)
  line L1402 (-150.1255, -72.8813) -> (-150.1783, -72.9682)
  line L1403 (-150.1783, -72.9682) -> (-150.239, -73.0493)
  line L1404 (-150.239, -73.0493) -> (-150.307, -73.1241)
  line L1405 (-150.307, -73.1241) -> (-150.3818, -73.1921)
  line L1406 (-150.3818, -73.1921) -> (-150.4629, -73.2528)
  line L1407 (-150.4629, -73.2528) -> (-150.5497, -73.3056)
  line L1408 (-150.5497, -73.3056) -> (-150.6418, -73.35)
  line L1409 (-150.6418, -73.35) -> (-150.7386, -73.3855)
  line L1410 (-150.7386, -73.3855) -> (-150.8395, -73.4114)
  line L1411 (-150.8395, -73.4114) -> (-150.9441, -73.4273)
  line L1412 (-150.9441, -73.4273) -> (-151.0517, -73.4333)
  line L1413 (-151.0517, -73.4333) -> (-154.4274, -73.4333)
  line L1414 (-154.4274, -73.4333) -> (-154.3752, -73.7192)
  line L1415 (-154.3752, -73.7192) -> (-154.3015, -73.9941)
  line L1416 (-154.3015, -73.9941) -> (-154.2073, -74.2569)
  line L1417 (-154.2073, -74.2569) -> (-154.0934, -74.5067)
  line L1418 (-154.0934, -74.5067) -> (-153.9608, -74.7424)
  line L1419 (-153.9608, -74.7424) -> (-153.8102, -74.963)
  line L1420 (-153.8102, -74.963) -> (-153.6426, -75.1674)
  line L1421 (-153.6426, -75.1674) -> (-153.4589, -75.3547)
  line L1422 (-153.4589, -75.3547) -> (-153.26, -75.5238)
  line L1423 (-153.26, -75.5238) -> (-153.0467, -75.6737)
  line L1424 (-153.0467, -75.6737) -> (-152.82, -75.8033)
  line L1425 (-152.82, -75.8033) -> (-152.5807, -75.9117)
  line L1426 (-152.5807, -75.9117) -> (-152.3297, -75.9978)
  line L1427 (-152.3297, -75.9978) -> (-152.068, -76.0606)
  line L1428 (-152.068, -76.0606) -> (-151.7963, -76.099)
  line L1429 (-151.7963, -76.099) -> (-151.5156, -76.112)
  line L1430 (-151.5156, -76.112) -> (-151.1789, -76.0985)
  line L1431 (-151.1789, -76.0985) -> (-150.8666, -76.0591)
  line L1432 (-150.8666, -76.0591) -> (-150.5778, -75.9956)
  line L1433 (-150.5778, -75.9956) -> (-150.3116, -75.9096)
  line L1434 (-150.3116, -75.9096) -> (-150.067, -75.8029)
  line L1435 (-150.067, -75.8029) -> (-149.8433, -75.6772)
  line L1436 (-149.8433, -75.6772) -> (-149.6394, -75.5342)
  line L1437 (-149.6394, -75.5342) -> (-149.4545, -75.3756)
  line L1438 (-149.4545, -75.3756) -> (-149.2876, -75.2032)
  line L1439 (-149.2876, -75.2032) -> (-149.1379, -75.0187)
  line L1440 (-149.1379, -75.0187) -> (-149.0044, -74.8237)
  line L1441 (-149.0044, -74.8237) -> (-148.8863, -74.6199)
  line L1442 (-148.8863, -74.6199) -> (-148.7827, -74.4092)
  line L1443 (-148.7827, -74.4092) -> (-148.6926, -74.1932)
  line L1444 (-148.6926, -74.1932) -> (-148.6151, -73.9737)
  line L1445 (-148.6151, -73.9737) -> (-148.5493, -73.7522)
  line L1446 (-148.5493, -73.7522) -> (-148.4944, -73.5307)
  line L1447 (-148.4944, -73.5307) -> (-148.4494, -73.3107)
  line L1448 (-148.4494, -73.3107) -> (-148.4134, -73.094)
  line L1449 (-148.4134, -73.094) -> (-148.3855, -72.8823)
  line L1450 (-148.3855, -72.8823) -> (-148.3504, -72.4808)
  line L1451 (-148.3504, -72.4808) -> (-148.3368, -72.1199)
  line L1452 (-148.3368, -72.1199) -> (-148.3376, -71.8133)
  line L1453 (-148.3376, -71.8133) -> (-148.3456, -71.5748)
  line L1454 (-148.3456, -71.5748) -> (-148.3536, -71.3569)
  line L1455 (-148.3536, -71.3569) -> (-148.3674, -71.0195)
  line L1456 (-148.3674, -71.0195) -> (-148.4086, -70.6952)
  line L1457 (-148.4086, -70.6952) -> (-148.4766, -70.385)
  line L1458 (-148.4766, -70.385) -> (-148.5709, -70.0901)
  line L1459 (-148.5709, -70.0901) -> (-148.6277, -69.9489)
  line L1460 (-148.6277, -69.9489) -> (-148.6909, -69.8119)
  line L1461 (-148.6909, -69.8119) -> (-148.7604, -69.6794)
  line L1462 (-148.7604, -69.6794) -> (-148.8362, -69.5514)
  line L1463 (-148.8362, -69.5514) -> (-148.9182, -69.4283)
  line L1464 (-148.9182, -69.4283) -> (-149.0063, -69.31)
  line L1465 (-149.0063, -69.31) -> (-149.1004, -69.1968)
  line L1466 (-149.1004, -69.1968) -> (-149.2005, -69.0888)
  line L1467 (-149.2005, -69.0888) -> (-149.3066, -68.9862)
  line L1468 (-149.3066, -68.9862) -> (-149.4185, -68.8891)
  line L1469 (-149.4185, -68.8891) -> (-149.5362, -68.7977)
  line L1470 (-149.5362, -68.7977) -> (-149.6596, -68.7121)
  line L1471 (-149.6596, -68.7121) -> (-149.7887, -68.6325)
  line L1472 (-149.7887, -68.6325) -> (-149.9234, -68.559)
  line L1473 (-149.9234, -68.559) -> (-150.0636, -68.4918)
  line L1474 (-150.0636, -68.4918) -> (-150.2093, -68.431)
  line L1475 (-150.2093, -68.431) -> (-150.3604, -68.3768)
  line L1476 (-150.3604, -68.3768) -> (-150.5168, -68.3293)
  line L1477 (-150.5168, -68.3293) -> (-150.6785, -68.2887)
  line L1478 (-150.6785, -68.2887) -> (-150.8454, -68.2552)
  line L1479 (-150.8454, -68.2552) -> (-151.0175, -68.2287)
  line L1480 (-151.0175, -68.2287) -> (-151.1946, -68.2097)
  line L1481 (-151.1946, -68.2097) -> (-151.3767, -68.1981)
  line L1482 (-151.3767, -68.1981) -> (-151.5638, -68.1941)
  line L1483 (-151.5638, -68.1941) -> (-151.5688, -68.2021)
  line L1484 (-151.5688, -68.2021) -> (-155.3855, -68.7888)
  line L1485 (-155.3855, -68.7888) -> (-155.5538, -68.8063)
  line L1486 (-155.5538, -68.8063) -> (-155.712, -68.8093)
  line L1487 (-155.712, -68.8093) -> (-155.8602, -68.7958)
  line L1488 (-155.8602, -68.7958) -> (-155.9982, -68.7684)
  line L1489 (-155.9982, -68.7684) -> (-156.1262, -68.728)
  line L1490 (-156.1262, -68.728) -> (-156.2441, -68.6756)
  line L1491 (-156.2441, -68.6756) -> (-156.3519, -68.6121)
  line L1492 (-156.3519, -68.6121) -> (-156.4497, -68.5385)
  line L1493 (-156.4497, -68.5385) -> (-156.5375, -68.4558)
  line L1494 (-156.5375, -68.4558) -> (-156.6152, -68.3649)
  line L1495 (-156.6152, -68.3649) -> (-156.6829, -68.2667)
  line L1496 (-156.6829, -68.2667) -> (-156.7406, -68.1623)
  line L1497 (-156.7406, -68.1623) -> (-156.7883, -68.0526)
  line L1498 (-156.7883, -68.0526) -> (-156.8261, -67.9386)
  line L1499 (-156.8261, -67.9386) -> (-156.8539, -67.8212)
  line L1500 (-156.8539, -67.8212) -> (-156.8717, -67.7015)
  line L1501 (-156.8717, -67.7015) -> (-156.8807, -67.5289)
  line L1502 (-156.8807, -67.5289) -> (-156.8702, -67.3645)
  line L1503 (-156.8702, -67.3645) -> (-156.8418, -67.2086)
  line L1504 (-156.8418, -67.2086) -> (-156.7966, -67.0611)
  line L1505 (-156.7966, -67.0611) -> (-156.7358, -66.9224)
  line L1506 (-156.7358, -66.9224) -> (-156.6607, -66.7925)
  line L1507 (-156.6607, -66.7925) -> (-156.5724, -66.6715)
  line L1508 (-156.5724, -66.6715) -> (-156.4722, -66.5597)
  line L1509 (-156.4722, -66.5597) -> (-156.3612, -66.4571)
  line L1510 (-156.3612, -66.4571) -> (-156.2408, -66.364)
  line L1511 (-156.2408, -66.364) -> (-156.112, -66.2805)
  line L1512 (-156.112, -66.2805) -> (-155.9761, -66.2068)
  line L1513 (-155.9761, -66.2068) -> (-155.8344, -66.143)
  line L1514 (-155.8344, -66.143) -> (-155.6879, -66.0892)
  line L1515 (-155.6879, -66.0892) -> (-155.538, -66.0457)
  line L1516 (-155.538, -66.0457) -> (-155.3858, -66.0126)
  line L1517 (-155.3858, -66.0126) -> (-151.5638, -65.4852)
  line L1518 (-151.5638, -65.4852) -> (-151.1178, -65.4952)
  line L1519 (-151.1178, -65.4952) -> (-150.6892, -65.5233)
  line L1520 (-150.6892, -65.5233) -> (-150.278, -65.5693)
  line L1521 (-150.278, -65.5693) -> (-149.8837, -65.6326)
  line L1522 (-149.8837, -65.6326) -> (-149.5063, -65.7125)
  line L1523 (-149.5063, -65.7125) -> (-149.1455, -65.8084)
  line L1524 (-149.1455, -65.8084) -> (-148.8011, -65.9197)
  line L1525 (-148.8011, -65.9197) -> (-148.4729, -66.0456)
  line L1526 (-148.4729, -66.0456) -> (-148.1606, -66.1855)
  line L1527 (-148.1606, -66.1855) -> (-147.864, -66.3389)
  line L1528 (-147.864, -66.3389) -> (-147.583, -66.5049)
  line L1529 (-147.583, -66.5049) -> (-147.3173, -66.6831)
  line L1530 (-147.3173, -66.6831) -> (-147.0666, -66.8727)
  line L1531 (-147.0666, -66.8727) -> (-146.8308, -67.0731)
  line L1532 (-146.8308, -67.0731) -> (-146.6097, -67.2837)
  line L1533 (-146.6097, -67.2837) -> (-146.403, -67.5037)
  line L1534 (-146.403, -67.5037) -> (-146.2105, -67.7326)
  line L1535 (-146.2105, -67.7326) -> (-146.032, -67.9697)
  line L1536 (-146.032, -67.9697) -> (-145.8673, -68.2144)
  line L1537 (-145.8673, -68.2144) -> (-145.7161, -68.4659)
  line L1538 (-145.7161, -68.4659) -> (-145.5783, -68.7237)
  line L1539 (-145.5783, -68.7237) -> (-145.4536, -68.9872)
  line L1540 (-145.4536, -68.9872) -> (-145.3418, -69.2555)
  line L1541 (-145.3418, -69.2555) -> (-145.2427, -69.5282)
  line L1542 (-145.2427, -69.5282) -> (-145.1561, -69.8046)
  line L1543 (-145.1561, -69.8046) -> (-145.0817, -70.0839)
  line L1544 (-145.0817, -70.0839) -> (-145.0194, -70.3657)
  line L1545 (-145.0194, -70.3657) -> (-144.9689, -70.6491)
  line L1546 (-144.9689, -70.6491) -> (-144.93, -70.9336)
  line L1547 (-144.93, -70.9336) -> (-144.9025, -71.2185)
  line L1548 (-144.9025, -71.2185) -> (-144.8861, -71.5032)
  line L1549 (-144.8861, -71.5032) -> (-144.8811, -71.7871)
  line L1550 (-144.8811, -71.7871) -> (-144.8881, -72.1621)
  line L1551 (-144.8881, -72.1621) -> (-144.9094, -72.529)
  line L1552 (-144.9094, -72.529) -> (-144.9448, -72.8877)
  line L1553 (-144.9448, -72.8877) -> (-144.9942, -73.2378)
  line L1554 (-144.9942, -73.2378) -> (-145.0573, -73.5791)
  line L1555 (-145.0573, -73.5791) -> (-145.1341, -73.9113)
  line L1556 (-145.1341, -73.9113) -> (-145.2244, -74.2342)
  line L1557 (-145.2244, -74.2342) -> (-145.328, -74.5476)
  line L1558 (-145.328, -74.5476) -> (-145.4448, -74.8511)
  line L1559 (-145.4448, -74.8511) -> (-145.5747, -75.1445)
  line L1560 (-145.5747, -75.1445) -> (-145.7175, -75.4276)
  line L1561 (-145.7175, -75.4276) -> (-145.873, -75.7002)